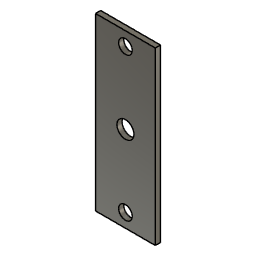
5D_Gambar F3Z_Aeroflow Brake Cooler (Autodesk Fusion 360 archive; units mm, degrees)
design "Mounting AeroFlow BrakeCooler v1[1]"
Autodesk Fusion 360 part; units mm, degrees
sketch "Sketch1" plane through (0, 0, 0) normal (0, 1, 0) x (1, 0, 0)
  line L0 (0, 0) -> (35, 0)
  line L1 (35, 0) -> (35, -100)
  line L2 (35, -100) -> (0, -100)
  line L3 (0, -100) -> (0, 0)
  line L4 (17.5, -100) -> (17.5, -92)
  circle A0 centre (17.5, -92) radius 4
  line L5 (17.5, 0) -> (17.5, -8)
  circle A1 centre (17.5, -8) radius 4
  line L6 (0, -50) -> (17.5, -50)
  circle A2 centre (17.5, -50) radius 5
  dimension "d1" = 35
  dimension "d2" = 100
  dimension "d3" = 8
  dimension "d4" = 8
  dimension "d5" = 8
  dimension "d6" = 8
  dimension "d7" = 10
  constraint horizontal L0
  constraint vertical L1
  constraint horizontal L2
  constraint vertical L3
  constraint coincident L0.start L3.end
  constraint midpoint L2 L4.start
  constraint perpendicular L2 L4
  constraint coincident L4.end A0.centre
  constraint midpoint L0 L5.start
  constraint perpendicular L0 L5
  constraint coincident L5.end A1.centre
  constraint midpoint L3 L6.start
  constraint perpendicular L4 L6
  constraint coincident L6.end A2.centre
  measures "d1" distance of L0.start L0.end
  measures "d2" distance of L0.end L1.end
  measures "d3" distance of L4.start L4.end
  measures "d4" diameter of A0
  measures "d5" distance of L5.start L5.end
  measures "d6" diameter of A1
  measures "d7" diameter of A2
extrude "Extrude1" add sketch "Sketch1" along normal blind 3

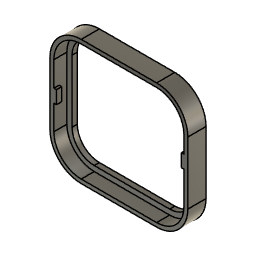
design "Cover Filter Bawah AeroFlow Brakecooler v1[1]"
Autodesk Fusion 360 part; units mm, degrees
sketch "Sketch1" plane through (0, 0, 0) normal (0, 1, 0) x (1, 0, 0)
  line L0 (0, 0) -> (53, 0)
  line L1 (53, 0) -> (53, -48)
  line L2 (53, -48) -> (0, -48)
  line L3 (0, -48) -> (0, 0)
  dimension "d1" = 48
  dimension "d2" = 53
  constraint horizontal L0
  constraint vertical L1
  constraint horizontal L2
  constraint vertical L3
  constraint coincident L0.start L3.end
  measures "d1" distance of L0.start L2.end
  measures "d2" distance of L0.start L0.end
extrude "Extrude1" add sketch "Sketch1" along normal blind 7
fillet "Fillet1" radius 12 3 edges at (0, 3.5, 48) (0, 3.5, 0) (53, 3.5, 0)
fillet "Fillet2" radius 12 1 edges at (53, 3.5, 48)
sketch "Sketch2" plane through (0, 0, 0) normal (0, -1, 0) x (1, 0, 0)
  arc A0 (53, 36) -> (41, 48) centre (41, 36) ccw
  line L0 (41, 48) -> (12, 48)
  arc A1 (12, 48) -> (0, 36) centre (12, 36) ccw
  line L1 (0, 36) -> (0, 12)
  arc A2 (0, 12) -> (12, 0) centre (12, 12) ccw
  line L2 (12, 0) -> (41, 0)
  arc A3 (41, 0) -> (53, 12) centre (41, 12) ccw
  line L3 (53, 12) -> (53, 36)
  line L4 (12, 1.5) -> (41, 1.5)
  arc A4 (41, 1.5) -> (51.5, 12) centre (41, 12) ccw
  line L5 (51.5, 12) -> (51.5, 36)
  arc A5 (51.5, 36) -> (41, 46.5) centre (41, 36) ccw
  line L6 (41, 46.5) -> (12, 46.5)
  arc A6 (12, 46.5) -> (1.5, 36) centre (12, 36) ccw
  line L7 (1.5, 36) -> (1.5, 12)
  arc A7 (1.5, 12) -> (12, 1.5) centre (12, 12) ccw
  dimension "d9" = -1.5
extrude "Extrude2" cut sketch "Sketch2" against normal blind 5 contours L4 A4 L5 A5 L6 A6 L7 A7
sketch "Sketch3" plane through (0, 7, 0) normal (0, 1, 0) x (-1, 0, 0)
  arc A0 (-41, 48) -> (-53, 36) centre (-41, 36) ccw
  line L0 (-53, 36) -> (-53, 12)
  arc A1 (-53, 12) -> (-41, 0) centre (-41, 12) ccw
  line L1 (-41, 0) -> (-12, 0)
  arc A2 (-12, 0) -> (0, 12) centre (-12, 12) ccw
  line L2 (0, 12) -> (0, 36)
  arc A3 (0, 36) -> (-12, 48) centre (-12, 36) ccw
  line L3 (-12, 48) -> (-41, 48)
  arc A4 (-41, 44.5) -> (-49.5, 36) centre (-41, 36) ccw
  line L4 (-49.5, 36) -> (-49.5, 12)
  arc A5 (-49.5, 12) -> (-41, 3.5) centre (-41, 12) ccw
  line L5 (-41, 3.5) -> (-12, 3.5)
  arc A6 (-12, 3.5) -> (-3.5, 12) centre (-12, 12) ccw
  line L6 (-3.5, 12) -> (-3.5, 36)
  arc A7 (-3.5, 36) -> (-12, 44.5) centre (-12, 36) ccw
  line L7 (-12, 44.5) -> (-41, 44.5)
  dimension "d12" = -3.5
extrude "Extrude3" cut sketch "Sketch3" against normal blind 2 contours A4 L4 A5 L5 A6 L6 A7 L7
sketch "Sketch4" plane through (1.5, 0, 0) normal (1, 0, 0) x (0, 1, 0)
  line L0 (0, 36) -> (0, 12)
  line L1 (0, 12) -> (5, 12)
  line L2 (5, 12) -> (5, 36)
  line L3 (5, 36) -> (0, 36)
  line L4 (0, 12) -> (0, 36)
  line L5 (0, 36) -> (0, 24)
  line L6 (2, 24) -> (2, 26.5)
  line L7 (2, 24) -> (2, 21.5)
  line L8 (2, 21.5) -> (0, 21.5)
  line L9 (0, 26.5) -> (2, 26.5)
  dimension "d15" = 2
  dimension "d16" = 2.5
  dimension "d17" = 2.5
  constraint coincident L0.start L3.end
  constraint midpoint L4 L5.end
  constraint coincident L4 L8.end
  constraint perpendicular L4 L8
  constraint coincident L5 L9.start
  measures "d15" distance of L5.end L6.start
  measures "d16" distance of L6.start L6.end
  measures "d17" distance of L6.start L7.end
extrude "Extrude4" add sketch "Sketch4" along normal blind 1 contours L0 L4 L5 L6 L7 L8 L9
sketch "Sketch5" plane through (51.5, 0, 0) normal (-1, 0, 0) x (0, -1, 0)
  line L0 (0, 12) -> (0, 36)
  line L1 (0, 36) -> (-5, 36)
  line L2 (-5, 36) -> (-5, 12)
  line L3 (-5, 12) -> (0, 12)
  line L4 (0, 36) -> (0, 12)
  line L5 (-2, 27) -> (-2, 29.5)
  line L6 (-2, 27) -> (-2, 24.5)
  line L7 (-2, 24.5) -> (0, 24.5)
  line L8 (0, 24.5) -> (0, 29.5)
  line L9 (-2, 29.5) -> (0, 29.5)
  dimension "d21" = 2.5
  dimension "d22" = 2.5
  constraint coincident L0 L7.end
  constraint perpendicular L0 L7
  constraint coincident L0 L8.end
  measures "d21" distance of L5.start L5.end
  measures "d22" distance of L5.start L6.end
extrude "Extrude5" add sketch "Sketch5" along normal blind 1 contours L0 L4 L5 L6 L7 L8 L9

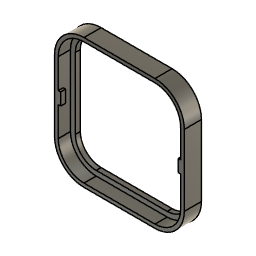
design "Cover Filter Atas AeroFlow Brakecooler v1[1]"
Autodesk Fusion 360 part; units mm, degrees
sketch "Sketch1" plane through (0, 0, 0) normal (0, 1, 0) x (1, 0, 0)
  line L0 (0, 0) -> (53, 0)
  line L1 (53, 0) -> (53, -53)
  line L2 (53, -53) -> (0, -53)
  line L3 (0, -53) -> (0, 0)
  dimension "d1" = 53
  dimension "d2" = 53
  constraint horizontal L0
  constraint vertical L1
  constraint horizontal L2
  constraint vertical L3
  constraint coincident L0.start L3.end
  measures "d1" distance of L0.start L2.end
  measures "d2" distance of L0.start L0.end
extrude "Extrude1" add sketch "Sketch1" along normal blind 7
fillet "Fillet1" radius 12 3 edges at (0, 3.5, 53) (0, 3.5, 0) (53, 3.5, 0)
fillet "Fillet2" radius 12 1 edges at (53, 3.5, 53)
sketch "Sketch2" plane through (0, 0, 0) normal (0, -1, 0) x (1, 0, 0)
  arc A0 (53, 41) -> (41, 53) centre (41, 41) ccw
  line L0 (41, 53) -> (12, 53)
  arc A1 (12, 53) -> (0, 41) centre (12, 41) ccw
  line L1 (0, 41) -> (0, 12)
  arc A2 (0, 12) -> (12, 0) centre (12, 12) ccw
  line L2 (12, 0) -> (41, 0)
  arc A3 (41, 0) -> (53, 12) centre (41, 12) ccw
  line L3 (53, 12) -> (53, 41)
  line L4 (12, 1.5) -> (41, 1.5)
  arc A4 (41, 1.5) -> (51.5, 12) centre (41, 12) ccw
  line L5 (51.5, 12) -> (51.5, 41)
  arc A5 (51.5, 41) -> (41, 51.5) centre (41, 41) ccw
  line L6 (41, 51.5) -> (12, 51.5)
  arc A6 (12, 51.5) -> (1.5, 41) centre (12, 41) ccw
  line L7 (1.5, 41) -> (1.5, 12)
  arc A7 (1.5, 12) -> (12, 1.5) centre (12, 12) ccw
  dimension "d9" = -1.5
extrude "Extrude2" cut sketch "Sketch2" against normal blind 5 contours L4 A4 L5 A5 L6 A6 L7 A7
sketch "Sketch3" plane through (0, 7, 0) normal (0, 1, 0) x (-1, 0, 0)
  arc A0 (-41, 53) -> (-53, 41) centre (-41, 41) ccw
  line L0 (-53, 41) -> (-53, 12)
  arc A1 (-53, 12) -> (-41, 0) centre (-41, 12) ccw
  line L1 (-41, 0) -> (-12, 0)
  arc A2 (-12, 0) -> (0, 12) centre (-12, 12) ccw
  line L2 (0, 12) -> (0, 41)
  arc A3 (0, 41) -> (-12, 53) centre (-12, 41) ccw
  line L3 (-12, 53) -> (-41, 53)
  arc A4 (-41, 49.5) -> (-49.5, 41) centre (-41, 41) ccw
  line L4 (-49.5, 41) -> (-49.5, 12)
  arc A5 (-49.5, 12) -> (-41, 3.5) centre (-41, 12) ccw
  line L5 (-41, 3.5) -> (-12, 3.5)
  arc A6 (-12, 3.5) -> (-3.5, 12) centre (-12, 12) ccw
  line L6 (-3.5, 12) -> (-3.5, 41)
  arc A7 (-3.5, 41) -> (-12, 49.5) centre (-12, 41) ccw
  line L7 (-12, 49.5) -> (-41, 49.5)
  dimension "d12" = -3.5
extrude "Extrude3" cut sketch "Sketch3" against normal blind 2 contours A4 L4 A5 L5 A6 L6 A7 L7
sketch "Sketch4" plane through (1.5, 0, 0) normal (1, 0, 0) x (0, 1, 0)
  line L0 (0, 41) -> (0, 12)
  line L1 (0, 12) -> (5, 12)
  line L2 (5, 12) -> (5, 41)
  line L3 (5, 41) -> (0, 41)
  line L4 (0, 12) -> (0, 41)
  line L5 (0, 41) -> (0, 26.5)
  line L6 (2, 26.5) -> (2, 29)
  line L7 (2, 26.5) -> (2, 24)
  line L8 (2, 24) -> (0, 24)
  line L9 (0, 29) -> (2, 29)
  dimension "d15" = 2
  dimension "d16" = 2.5
  dimension "d17" = 2.5
  constraint coincident L0.start L3.end
  constraint midpoint L4 L5.end
  constraint coincident L4 L8.end
  constraint perpendicular L4 L8
  constraint coincident L5 L9.start
  measures "d15" distance of L5.end L6.start
  measures "d16" distance of L6.start L6.end
  measures "d17" distance of L6.start L7.end
extrude "Extrude4" add sketch "Sketch4" along normal blind 1 contours L0 L4 L5 L6 L7 L8 L9
sketch "Sketch5" plane through (51.5, 0, 0) normal (-1, 0, 0) x (0, -1, 0)
  line L0 (0, 12) -> (0, 41)
  line L1 (0, 41) -> (-5, 41)
  line L2 (-5, 41) -> (-5, 12)
  line L3 (-5, 12) -> (0, 12)
  line L4 (0, 41) -> (0, 12)
  line L5 (-2, 27) -> (-2, 29.5)
  line L6 (-2, 27) -> (-2, 24.5)
  line L7 (-2, 24.5) -> (0, 24.5)
  line L8 (0, 24.5) -> (0, 29.5)
  line L9 (-2, 29.5) -> (0, 29.5)
  dimension "d21" = 2.5
  dimension "d22" = 2.5
  constraint coincident L0 L7.end
  constraint perpendicular L0 L7
  constraint coincident L0 L8.end
  measures "d21" distance of L5.start L5.end
  measures "d22" distance of L5.start L6.end
extrude "Extrude5" add sketch "Sketch5" along normal blind 1 contours L0 L4 L5 L6 L7 L8 L9
